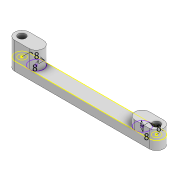
# Autodesk Inventor part: Part_9
Saved by Autodesk Inventor 2022 (Build 260153000, 153)
## iProperties
Created: 2022-04-21
Part Number: Part_9
Material: Generic
Document SubType Name: Modeling
Designer: dell
Density: 1 g/cm^3
Appearance: Default
Author: dell
Autodesk Inventor part; units mm, degrees
ref_plane "YZ Plane" through (0, 0, 0) normal (1, 0, 0) x (0, 1, 0)
ref_plane "XZ Plane" through (0, 0, 0) normal (0, 1, 0) x (-1, 0, 0)
ref_plane "XY Plane" through (0, 0, 0) normal (0, 0, 1) x (1, 0, 0)
sketch "Sketch1" plane through (0, 0, 0) normal (0, 1, 0) x (-1, 0, 0)
  line L0 (0, 0) -> (-75.105, 0) construction
  line L1 (0, 4) -> (-75.105, 4)
  line L2 (-75.105, -4) -> (0, -4)
  arc A0 (0, -4) -> (0, 4) centre (0, 0) ccw
  arc A1 (-75.105, 4) -> (-75.105, -4) centre (-75.105, 0) ccw
  circle A2 centre (0, 0) radius 2.1
  circle A3 centre (-75.105, 0) radius 2.1
  point P0 (-37.5525, 0)
  dimension "d0" = 75.105
  dimension "d1" = 8
  dimension "d2" = 4.2
  dimension "d10" = 4.2
  constraints: 8 end point, 4 centre point, 4 point on circle, 4 tangent, 2 coincident, 1 horizontal, 1 midpoint, 1 parallel
  measures "d0" distance of L0.end L0.start
  measures "d1" distance between parallel lines of L1 L2
  measures "d2" diameter of A2
  measures "d10" diameter of A3
extrude "Extrusion1" add sketch "Sketch1" along normal blind 5
sketch "Sketch4" plane through (0, 5, 0) normal (0, 1, 0) x (1, 0, 0)
  circle A0 centre (8, 0) radius 4
  circle A1 centre (67.105, 0) radius 4
  arc A2 (75.105, -4) -> (75.105, 4) centre (75.105, 0) ccw projected
  line L0 (75.105, 4) -> (0, 4) projected
  arc A3 (0, 4) -> (0, -4) centre (0, 0) ccw projected
  line L1 (0, -4) -> (75.105, -4) projected
  circle A4 centre (75.105, 0) radius 2.1 projected
  circle A5 centre (0, 0) radius 2.1 projected
  point P0 (8, -4)
  point P1 (8, 4)
  point P2 (67.105, 4)
  point P3 (67.105, -4)
  dimension "d30" = 8
  dimension "d31" = 8
  dimension "d32" = 8
  dimension "d33" = 8
  constraints: 2 centre point
  measures "d30" diameter of A0
  measures "d31" diameter of A1
  measures "d32" distance of point (0, 0) A0.centre
  measures "d33" distance of A2.centre A1.centre
extrude "Extrusion7" add sketch "Sketch4" along normal blind 10 contours A0 | A0 L1 A3 L0
extrude "Extrusion8" add sketch "Sketch4" along normal blind 5 contours L0 A2 L1 A1 | A1
body "Solid1"
